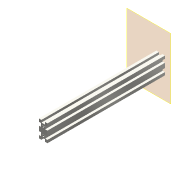
# Autodesk Inventor part: Neje_Aluminium_Slide_X
Saved by Autodesk Inventor 2019.4 (Build 234330000, 330)
## iProperties
Created: 2021-04-08
Part Number: Neje_Aluminium_Slide_X
Material: Generic
Document SubType Name: Modeling
Designer: diederichbenedict
Density: 1 g/cm^3
Appearance: Silver
Author: diederichbenedict
Autodesk Inventor part; units mm, degrees
ref_plane "YZ Plane" through (0, 0, 0) normal (1, 0, 0) x (0, 1, 0)
ref_plane "XZ Plane" through (0, 0, 0) normal (0, 1, 0) x (-1, 0, 0)
ref_plane "Work Plane1" through (0, 0, 0) normal (0, 0, 1) x (1, 0, 0)
sketch "Sketch1" plane through (0, 0, 0) normal (0, 0, 1) x (1, 0, 0)
  circle A0 centre (-23.32, -39.075) radius 2.355 projected
  circle A1 centre (-23.32, 39.075) radius 2.355 projected
  circle A2 centre (20.82, -6.975) radius 2 projected
  circle A3 centre (20.82, 7.075) radius 2 projected
  line L0 (32.82, 48.575) -> (-32.82, 48.575) projected
  arc A4 (-32.82, 48.575) -> (-34.82, 46.575) centre (-32.82, 46.575) ccw projected
  line L1 (-34.82, 46.575) -> (-34.82, -46.575) projected
  arc A5 (-34.82, -46.575) -> (-32.82, -48.575) centre (-32.82, -46.575) ccw projected
  line L2 (-32.82, -48.575) -> (32.82, -48.575) projected
  arc A6 (32.82, -48.575) -> (34.82, -46.575) centre (32.82, -46.575) ccw projected
  line L3 (34.82, -46.575) -> (34.82, 46.575) projected
  arc A7 (34.82, 46.575) -> (32.82, 48.575) centre (32.82, 46.575) ccw projected
  line L4 (13.32, -15) -> (28.32, 15) construction
  line L5 (28.32, -15) -> (13.32, 15) construction
  line L6 (32.32, 10.075) -> (24.32, 10.075)
  line L7 (24.32, 10.075) -> (24.32, 4.075)
  line L8 (24.32, 4.075) -> (32.32, 4.075)
  line L9 (32.32, 4.075) -> (32.32, 10.075)
  line L10 (32.32, 10.075) -> (24.32, 4.075) construction
  line L11 (24.32, 10.075) -> (32.32, 4.075) construction
  line L12 (32.32, -3.975) -> (24.32, -3.975)
  line L13 (24.32, -3.975) -> (24.32, -9.975)
  line L14 (24.32, -9.975) -> (32.32, -9.975)
  line L15 (32.32, -9.975) -> (32.32, -3.975)
  line L16 (32.32, -3.975) -> (24.32, -9.975) construction
  line L17 (24.32, -3.975) -> (32.32, -9.975) construction
  line L18 (9.32, 4.075) -> (17.32, 4.075)
  line L19 (17.32, 4.075) -> (17.32, 10.075)
  line L20 (17.32, 10.075) -> (9.32, 10.075)
  line L21 (9.32, 10.075) -> (9.32, 4.075)
  line L22 (9.32, 4.075) -> (17.32, 10.075) construction
  line L23 (17.32, 4.075) -> (9.32, 10.075) construction
  line L24 (9.32, -9.975) -> (17.32, -9.975)
  line L25 (17.32, -9.975) -> (17.32, -3.975)
  line L26 (17.32, -3.975) -> (9.32, -3.975)
  line L27 (9.32, -3.975) -> (9.32, -9.975)
  line L28 (9.32, -9.975) -> (17.32, -3.975) construction
  line L29 (17.32, -9.975) -> (9.32, -3.975) construction
  line L30 (23.82, 19) -> (17.82, 19)
  line L31 (17.82, 19) -> (17.82, 11)
  line L32 (17.82, 11) -> (23.82, 11)
  line L33 (23.82, 11) -> (23.82, 19)
  line L34 (23.82, 19) -> (17.82, 11) construction
  line L35 (17.82, 19) -> (23.82, 11) construction
  line L36 (17.82, -19) -> (23.82, -19)
  line L37 (23.82, -19) -> (23.82, -11)
  line L38 (23.82, -11) -> (17.82, -11)
  line L39 (17.82, -11) -> (17.82, -19)
  line L40 (17.82, -19) -> (23.82, -11) construction
  line L41 (23.82, -19) -> (17.82, -11) construction
  line L42 (28.32, 15) -> (23.82, 15)
  line L43 (17.82, 15) -> (13.32, 15)
  line L44 (28.32, 10.075) -> (28.32, 15)
  line L45 (28.32, -15) -> (28.32, -9.975)
  line L46 (28.32, -3.975) -> (28.32, 4.075)
  line L47 (13.32, -15) -> (17.82, -15)
  line L48 (23.82, -15) -> (28.32, -15)
  line L49 (13.32, -9.975) -> (13.32, -15)
  line L50 (13.32, 15) -> (13.32, 10.075)
  line L51 (13.32, 4.075) -> (13.32, -3.975)
  point P0 (0, 0)
  point P1 (20.82, 0)
  dimension "d0" = 15
  dimension "d1" = 30
  dimension "d2" = 8
  dimension "d3" = 6
  dimension "d4" = 6
  dimension "d5" = 8
  dimension "d6" = 6
  dimension "d7" = 8
  dimension "d8" = 6
  dimension "d9" = 8
  constraints: 96 end point, 26 midpoint, 25 parallel, 12 perpendicular, 8 horizontal, 4 point on line
  measures "d0" distance of L5.end L4.end
  measures "d1" distance of L4.end L5.start
  measures "d2" distance of L8.end L7.end
  measures "d3" distance of L7.end L6.end
  measures "d4" distance of L13.end L12.end
  measures "d5" distance of L20.end L19.end
  measures "d6" distance of L32.end L31.end
  measures "d7" distance of L31.end L30.end
  measures "d8" distance of L38.end L37.end
  measures "d9" distance of L37.end L36.end
ref_plane "Work Plane2" through (-34.82, -48.575, 205.34) normal (0, 0, -1) x (0, 1, 0)
extrude "Extrusion1" add sketch "Sketch1" along normal up to surface (205.34 mm away) contours L6 L7 L8 L46 L12 L13 L14 L45 L48 L37 L38 L39 L47 L49 L24 L25 L26 L51 L18 L19 L20 L50 L43 L31 L32 L33 L42 L44
body "Solid1"
